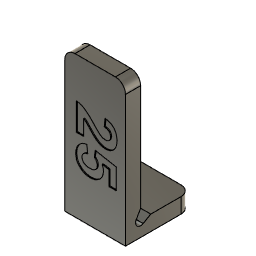
25mm 1515 Jig v2 (Autodesk Fusion 360 design; units mm, degrees)
Autodesk Fusion 360 part; units mm, degrees
note: some values were not read from the file. Set by a fixed rule: which sketch regions a step uses.
sketch "Sketch1" plane through (0, 0, 0) normal (1, 0, 0) x (0, 1, 0)
  line L0 (0, 0) -> (10, 0)
  line L1 (10, 0) -> (10, -3)
  line L2 (10, -3) -> (-3, -3)
  line L3 (-3, -3) -> (-3, 25)
  line L4 (-3, 25) -> (0, 25)
  line L5 (0, 25) -> (0, 0)
  circle A0 centre (0, 0) radius 1
  dimension "d1" = 25
  dimension "d2" = 10
  dimension "d3" = 3
  dimension "d4" = 3
  dimension "d5" = 2
  constraint coincident L0.start L5.end
  constraint horizontal L0
  constraint perpendicular L0 L1
  constraint perpendicular L1 L2
  constraint perpendicular L2 L3
  constraint perpendicular L3 L4
  constraint vertical L5
  measures "d1" distance of L0 L4
  measures "d2" distance of L0.start L0.end
  measures "d3" distance of L3.end L4.end
  measures "d4" distance of L0.end L1.end
  measures "d5" diameter of A0
extrude "Extrude1" add sketch "Sketch1" along normal blind 12 contours L0 L1 L2 L3 L4 L5 A0
chamfer "Chamfer1" distance 1 angle 45 2 edges at (6, 0, 1) (6, 1, 0)
sketch "Sketch2" plane through (0, 0, 0) normal (0, 1, 0) x (-1, 0, 0)
  line L0 (0, 2) -> (0, 25)
  line L1 (0, 25) -> (-12, 25)
  line L2 (-12, 25) -> (-12, 2)
  line L3 (-6, 25) -> (-6, -16.1804) construction
  line L4 (-7.3, 25) -> (-4.7, 25)
  line L5 (-4.7, 25) -> (-4.7, 2)
  line L6 (-4.7, 2) -> (-7.3, 2)
  line L7 (-7.3, 2) -> (-7.3, 25)
  line L8 (-12, 2) -> (0, 2)
  dimension "d8" = 2.6
  constraint midpoint L1 L3.start
  constraint horizontal L4
  constraint vertical L5
  constraint horizontal L6
  constraint vertical L7
  constraint coincident L1 L4.start
  constraint coincident L6.end L8
  measures "d8" distance of L5 L7
extrude "Extrude2" add sketch "Sketch2" along normal blind 1.2 contours L1 L4 L5 L6 L7 L8
chamfer "Chamfer2" distance 1.2 angle 45 2 edges at (6, 1.2, 2) (6, 1.2, 25)
fillet "Fillet1" radius 2 4 edges at (12, -1.5, 25) (0, -1.5, 25) (12, 10, -1.5) (0, 10, -1.5)
sketch "Sketch3" plane through (0, -3, 0) normal (0, -1, 0) x (1, 0, 0)
  arc A0 (2, 25) -> (0, 23) centre (2, 23) ccw
  line L0 (0, 23) -> (0, -3)
  line L1 (0, -3) -> (12, -3)
  line L2 (12, -3) -> (12, 23)
  arc A1 (12, 23) -> (10, 25) centre (10, 23) ccw
  line L3 (10, 25) -> (2, 25)
  line L4 (-1.1947, 17.0511) -> (-1.1947, 8.6202) construction
  line L5 (-1.1947, 8.6202) -> (10.2961, 8.6202) construction
  line L6 (10.2961, 8.6202) -> (10.2961, 17.0511) construction
  line L7 (10.2961, 17.0511) -> (-1.1947, 17.0511) construction
  dimension "d15" = 8
  text T0 "25" font "Arial" height 8 bold align left top in box 8.4309 x 11.4908 at (-1.1947, 17.0511) x (0, -1) y (1, 0) spacing 1
extrude "Extrude3" cut sketch "Sketch3" against normal blind 0.2 text T0
